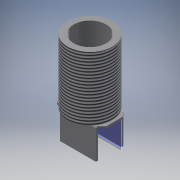
# Autodesk Inventor part: SPDT Toggle Switch Treaded Tube
Saved by Autodesk Inventor 2016 (Build 200138000, 138)
## iProperties
Created: 2011-11-07
Part Number: SPDT Toggle Switch Treaded Tube
Document SubType Name: Modeling
Designer: sdarley
Density: 1 g/cm^3
Material: Generic
Appearance: Polished Brushed
Author: sdarley
Autodesk Inventor part; units mm, degrees
ref_plane "YZ Plane" through (0, 0, 0) normal (1, 0, 0) x (0, 1, 0)
ref_plane "XZ Plane" through (0, 0, 0) normal (0, 1, 0) x (-1, 0, 0)
ref_plane "XY Plane" through (0, 0, 0) normal (0, 0, 1) x (1, 0, 0)
sketch "Sketch1" plane through (0, 0, 0) normal (0, 0, 1) x (1, 0, 0)
  line L0 (-0.5, 7) -> (-1.725, 7) projected
  line L1 (-13, 0.5) -> (-13, 6.5) projected
  line L2 (-11.275, 0) -> (-12.5, 0) projected
  line L3 (0, 0.5) -> (0, 6.5) projected
  arc A0 (0, 6.5) -> (-0.5, 7) centre (-0.5, 6.5) ccw projected
  line L4 (-1.725, 7) -> (-1.725, 6.5) projected
  line L5 (-1.725, 6.5) -> (-11.275, 6.5) projected
  line L6 (-11.275, 6.5) -> (-11.275, 7) projected
  arc A1 (-12.5, 7) -> (-13, 6.5) centre (-12.5, 6.5) ccw projected
  arc A2 (-13, 0.5) -> (-12.5, 0) centre (-12.5, 0.5) ccw projected
  line L7 (-11.275, 0) -> (-11.275, 0.5) projected
  line L8 (-11.275, 0.5) -> (-1.725, 0.5) projected
  line L9 (-1.725, 0.5) -> (-1.725, 0) projected
  line L10 (-0.5, 0) -> (-1.725, 0) projected
  arc A3 (-0.5, 0) -> (0, 0.5) centre (-0.5, 0.5) ccw projected
  line L11 (-13, 6.7) -> (0, 6.7)
  line L12 (0, 6.7) -> (0, 0.3)
  line L13 (0, 0.3) -> (-13, 0.3)
  line L14 (-13, 0.3) -> (-13, 6.7)
  line L15 (-11.275, 7) -> (-12.5, 7) projected
  dimension "d13" = 0.3
  dimension "d15" = 0.3
  constraints: 8 end point, 2 parallel, 1 horizontal, 1 perpendicular, 1 point on line
  measures "d13" distance between parallel lines of L0 L11
  measures "d15" distance between parallel lines of L2 L13
extrude "Extrusion3" add sketch "Sketch1" along normal blind 0.5 contours L11 L12 A0 | A0 L3 A3 L13 L9 L8 L7 A2 L1 A1 L11 L6 L5 L4 | L4 L5 L6 L11 | L12 L13 A3 | A1 L14 L11 | L13 L7 L8 L9 | A2 L13 L14
sketch "Sketch2" plane through (0, 0, 0.5) normal (0, 0, 1) x (1, 0, 0)
  circle A0 centre (-6.5, 3.5) radius 5.9
  circle A1 centre (-6.5, 3.5) radius 4.3
  point P0 (0, 0)
  dimension "d3" = 11.8
  dimension "d5" = 8.6
  constraints: 2 centre point, 1 coincident
  measures "d3" diameter of A0
  measures "d5" diameter of A1
extrude "Extrusion2" add sketch "Sketch2" along normal blind 16.8 separate body
thread "Thread1" size "M12x0.75" class "6g" standard "ISO Metric profile" full length
chamfer "Chamfer1" distance 1 angle 45 4 edges at (-13, 0.3, 0.25) (0, 0.3, 0.25) (0, 6.7, 0.25) (-13, 6.7, 0.25)
sketch "Sketch3" plane through (-12, 0.3, 0) normal (0, -1, 0) x (1, 0, 0)
  line L0 (11, 0.5) -> (0, 0.5) projected
  line L1 (1.225, -8) -> (1.225, 0) projected
  line L2 (10.775, 0) -> (10.775, -8) projected
  line L3 (1.225, 0.5) -> (10.775, 0.5)
  line L4 (10.775, 0.5) -> (10.775, -7.5)
  line L5 (10.775, -7.5) -> (1.225, -7.5)
  line L6 (1.225, -7.5) -> (1.225, 0.5)
  point P0 (12, 0)
  dimension "d18" = 8
  constraints: 8 end point, 2 parallel, 2 point on line, 1 horizontal, 1 perpendicular
  measures "d18" distance between parallel lines of L3 L5
extrude "Extrusion4" add sketch "Sketch3" along normal blind 0.5 bodies 1
ref_plane "Work Plane1" through (-11.275, 6.5, 0) normal (0, 1, 0) x (-1, 0, 0)
sketch "Sketch4" plane through (-11.275, 6.5, 0) normal (0, 1, 0) x (-1, 0, 0)
  line L0 (-0.5, -7.5) -> (-10.05, -7.5) projected
  line L1 (-9.55, -8) -> (-9.55, 0) projected
  line L2 (0, 0) -> (0, -8) projected
  line L3 (-0.5, 0) -> (-0.5, 0.5) projected
  line L4 (-10.05, 0.5) -> (-10.05, 0) projected
  line L5 (0.725, 0.5) -> (-10.275, 0.5) projected
  line L6 (-10.05, 0.5) -> (-0.5, 0.5)
  line L7 (-0.5, 0.5) -> (-0.5, -7.5)
  line L8 (-0.5, -7.5) -> (-10.05, -7.5)
  line L9 (-10.05, -7.5) -> (-10.05, 0.5)
  point P0 (-11.275, 0)
  constraints: 8 end point, 2 parallel, 1 horizontal, 1 perpendicular
extrude "Extrusion5" add sketch "Sketch4" along normal blind 0.5 bodies 1
fillet "Fillet1" radius 0.5 2 edges at (-6, 7, 0.5) (-6, -0.2, 0.5)
equation "\"d15\" = d13"
body "Solid1"
body "Solid2"
